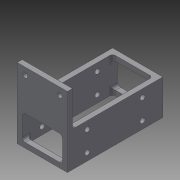
# Autodesk Inventor part: tubing_alignment_arm[2]
Saved by Autodesk Inventor 2015 (Build 190159000, 159)
## iProperties
Created: 2017-04-13
Part Number: tubing_alignment_arm[2]
Material: Generic
Document SubType Name: Modeling
Designer: Guy
Density: 1 g/cm^3
Appearance: Default
Author: Guy
Autodesk Inventor part; units mm, degrees
ref_plane "YZ Plane" through (0, 0, 0) normal (1, 0, 0) x (0, 1, 0)
ref_plane "XZ Plane" through (0, 0, 0) normal (0, 1, 0) x (-1, 0, 0)
ref_plane "XY Plane" through (0, 0, 0) normal (0, 0, 1) x (1, 0, 0)
sketch "Sketch1" plane through (0, 0, 0) normal (0, 0, 1) x (1, 0, 0)
  line L0 (0, 0) -> (50, 0)
  line L1 (50, 0) -> (50, 70)
  line L2 (50, 70) -> (0, 70)
  line L3 (0, 70) -> (0, 0)
  dimension "d0" = 50
  dimension "d1" = 70
  constraints: 8 end point, 2 parallel, 1 horizontal, 1 perpendicular
  measures "d0" distance of L0.start L0.end
  measures "d1" distance of L2.end L0.start
extrude "Extrusion1" add sketch "Sketch1" along normal blind 5
sketch "Sketch2" plane through (0, 0, 5) normal (0, 0, 1) x (1, 0, 0)
  circle A0 centre (7.825, 7) radius 2.5
  circle A1 centre (42.175, 7) radius 2.5
  line L0 (0, 0) -> (50, 0) projected
  line L1 (50, 0) -> (50, 70) projected
  line L2 (50, 70) -> (0, 70) projected
  line L3 (0, 70) -> (0, 0) projected
  dimension "d4" = 34.35
  dimension "d5" = 5
  dimension "d6" = 5
  dimension "d7" = 50
  dimension "d8" = 7.825
  dimension "d9" = 7
  dimension "d10" = 7
  constraints: 2 centre point
  measures "d4" distance of A1.centre A0.centre
  measures "d5" diameter of A0
  measures "d6" diameter of A1
  measures "d7" distance of L0.start L0.end
  measures "d8" distance from line of L1 A1.centre
  measures "d9" distance from line of L0 A1.centre
  measures "d10" distance from line of L0 A0.centre
extrude "Extrusion2" cut sketch "Sketch2" against normal up to next contours A0 | A1
sketch "Sketch3" plane through (0, 0, 5) normal (0, 0, 1) x (1, 0, 0)
  circle A0 centre (7.825, 7) radius 2.5 projected
  circle A1 centre (42.175, 7) radius 2.5 projected
  line L0 (0, 0) -> (50, 0) projected
  line L1 (50, 0) -> (50, 70) projected
  line L2 (50, 70) -> (0, 70) projected
  line L3 (0, 70) -> (0, 0) projected
  line L4 (0, 70) -> (5, 70)
  line L5 (5, 70) -> (5, 35)
  line L6 (5, 35) -> (0, 35)
  line L7 (0, 35) -> (0, 70)
  line L8 (50, 70) -> (45, 70)
  line L9 (45, 70) -> (45, 35)
  line L10 (45, 35) -> (50, 35)
  line L11 (50, 35) -> (50, 70)
  dimension "d13" = 5
  dimension "d14" = 5
  dimension "d15" = 35
  constraints: 16 end point, 4 parallel, 2 horizontal, 2 perpendicular, 1 point on line
  measures "d13" distance between parallel lines of L9 L1
  measures "d14" distance between parallel lines of L3 L5
  measures "d15" distance between parallel lines of L6 L2
extrude "Extrusion3" add sketch "Sketch3" along normal blind 90 contours L3 L2 L5 L6 | L10 L9 L2 L1
sketch "Sketch4" plane through (50, 0, 0) normal (1, 0, 0) x (0, 0, -1)
  line L0 (0, 0) -> (0, 70) projected
  line L1 (0, 70) -> (-95, 70) projected
  line L2 (-95, 35) -> (-95, 70) projected
  line L3 (-5, 35) -> (-95, 35) projected
  line L4 (-5, 0) -> (-5, 35) projected
  line L5 (0, 0) -> (-5, 0) projected
  circle A0 centre (-20, 62.5) radius 2.5
  circle A1 centre (-20, 42.5) radius 2.5
  circle A2 centre (-75, 62.5) radius 2.5
  circle A3 centre (-75, 42.5) radius 2.5
  point P0 (0, 0)
  dimension "d18" = 5
  dimension "d19" = 5
  dimension "d20" = 20
  dimension "d21" = 5
  dimension "d22" = 5
  dimension "d23" = 35
  dimension "d24" = 20
  dimension "d26" = 7.5
  dimension "d27" = 55
  dimension "d28" = 55
  dimension "d31" = 7.5
  dimension "d42" = 20
  dimension "d43" = 20
  constraints: 4 centre point
  measures "d18" diameter of A0
  measures "d19" diameter of A1
  measures "d20" distance of A1.centre A0.centre
  measures "d21" diameter of A2
  measures "d22" diameter of A3
  measures "d23" distance between parallel lines of L3 L1
  measures "d24" distance of A3.centre A2.centre
  measures "d26" distance from line of A2.centre L1
  measures "d27" distance of A0.centre A2.centre
  measures "d28" distance of A3.centre A1.centre
  measures "d31" distance from line of A0.centre L1
  measures "d42" distance from line of L0 A0.centre
  measures "d43" distance from line of L0 A1.centre
extrude "Extrusion4" cut sketch "Sketch4" against normal through all contours A0 | A1 | A2 | A3
sketch "Sketch5" plane through (5, 35, 5) normal (1, 0, 0) x (0, 0, -1)
  circle A0 centre (-70, 27.5) radius 2.5 projected
  circle A1 centre (-15, 27.5) radius 2.5 projected
  circle A2 centre (-15, 7.5) radius 2.5 projected
  circle A3 centre (-70, 7.5) radius 2.5 projected
  line L0 (0, 35) -> (0, 0) projected
  line L1 (0, 35) -> (-90, 35) projected
  line L2 (-90, 0) -> (-90, 35) projected
  line L3 (0, 0) -> (-90, 0) projected
  line L4 (0, 0) -> (-90, 0) projected
  line L5 (-90, 35) -> (-85, 35)
  line L6 (-85, 35) -> (-85, 0)
  line L7 (-85, 0) -> (-90, 0)
  line L8 (-90, 0) -> (-90, 35)
  point P0 (5, -35)
  dimension "d34" = 5
  constraints: 8 end point, 2 parallel, 1 horizontal, 1 perpendicular, 1 point on line
  measures "d34" distance between parallel lines of L2 L6
extrude "Extrusion5" add sketch "Sketch5" along normal up to next contours L6 L3 L2 L1
sketch "Sketch6" plane through (0, 0, 95) normal (0, 0, 1) x (1, 0, 0)
  line L0 (45, 35) -> (45, 70) projected
  line L1 (45, 70) -> (5, 70) projected
  line L2 (5, 70) -> (5, 35) projected
  line L3 (5, 35) -> (0, 35) projected
  line L4 (0, 35) -> (0, 0) projected
  line L5 (0, 0) -> (50, 0) projected
  line L6 (50, 0) -> (50, 35) projected
  line L7 (50, 35) -> (45, 35) projected
  circle A0 centre (7.825, 7) radius 2.5 projected
  circle A1 centre (42.175, 7) radius 2.5 projected
  line L8 (50, 70) -> (0, 70) projected
  line L9 (0, 70) -> (0, 35) projected
  line L10 (0, 35) -> (50, 35) projected
  line L11 (50, 35) -> (50, 70) projected
  line L12 (5, 65) -> (45, 65)
  line L13 (45, 65) -> (45, 40)
  line L14 (45, 40) -> (5, 40)
  line L15 (5, 40) -> (5, 65)
  dimension "d37" = 5
  dimension "d38" = 5
  constraints: 8 end point, 2 parallel, 2 point on line, 1 horizontal, 1 perpendicular
  measures "d37" distance between parallel lines of L12 L1
  measures "d38" distance between parallel lines of L10 L14
extrude "Extrusion6" cut sketch "Sketch6" against normal through all contours L14 L2 L12 L0
fillet "Fillet1" radius 3 18 edges at (47.5, 35, 5) (45, 37.5, 5) (2.5, 35, 5) (5, 37.5, 5) (5, 65, 2.5) (5, 67.5, 5) (5, 65, 92.5) (5, 67.5, 90) (45, 67.5, 5) (45, 65, 2.5) (45, 65, 92.5) (45, 67.5, 90) (45, 40, 2.5) (5, 40, 2.5) (45, 40, 92.5) (45, 37.5, 90) (5, 40, 92.5) (5, 37.5, 90)
equation "\"d8\" = -0.5 * d4 + 0.5 * d7"
equation "\"d10\" = d9"
equation "\"d13\" = d14"
equation "\"d26\" = -0.5 * d24 + 0.5 * d23"
equation "\"d28\" = d27"
equation "\"d31\" = d26"
equation "\"d43\" = d42"
body "Solid1"
